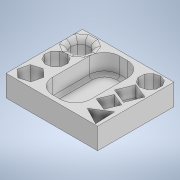
# Autodesk Inventor part: Dice Tower Base
Saved by Autodesk Inventor 2022 (Build 260153000, 153)
## iProperties
Created: 2022-07-25
Part Number: Dice Tower Base
Material: Generic
Document SubType Name: Modeling
Designer: dech3
Density: 1 g/cm^3
Appearance: Default
Author: dech3
Autodesk Inventor part; units mm, degrees
ref_plane "YZ Plane" through (0, 0, 0) normal (1, 0, 0) x (0, 1, 0)
ref_plane "XZ Plane" through (0, 0, 0) normal (0, 1, 0) x (-1, 0, 0)
ref_plane "XY Plane" through (0, 0, 0) normal (0, 0, 1) x (1, 0, 0)
sketch "Sketch1" plane through (0, 0, 0) normal (0, 1, 0) x (-1, 0, 0)
  line L0 (60, -50) -> (-60, -50)
  line L1 (-60, -50) -> (-60, 50)
  line L2 (-60, 50) -> (60, 50)
  line L3 (60, 50) -> (60, -50)
  point P0 (0, 0)
  dimension "d0" = 120
  dimension "d1" = 100
  dimension "d2" = 60
  dimension "d3" = 50
  constraints: 8 end point, 2 parallel, 1 horizontal, 1 perpendicular
  measures "d0" distance between parallel lines of L1 L3
  measures "d1" distance between parallel lines of L2 L0
  measures "d2" distance from line of point (0, 0) L1
  measures "d3" distance from line of point (0, 0) L0
extrude "Extrusion1" add sketch "Sketch1" along normal blind 28
sketch "Sketch2" plane through (0, 28, 0) normal (0, 1, 0) x (1, 0, 0)
  line L0 (-25, 44) -> (25, 44)
  line L1 (25, 44) -> (25, -44)
  line L2 (25, -44) -> (-25, -44)
  line L3 (-25, -44) -> (-25, 44)
  line L4 (60, 50) -> (-60, 50) projected
  line L5 (-60, -50) -> (60, -50) projected
  line L6 (60, -50) -> (60, 50) projected
  line L7 (-60, 50) -> (-60, -50) projected
  dimension "d20" = 6
  dimension "d21" = 6
  dimension "d22" = 35
  dimension "d23" = 35
  constraints: 8 end point, 2 parallel, 1 horizontal, 1 perpendicular
  measures "d20" distance between parallel lines of L0 L4
  measures "d21" distance between parallel lines of L5 L2
  measures "d22" distance between parallel lines of L1 L6
  measures "d23" distance between parallel lines of L7 L3
extrude "Extrusion2" cut sketch "Sketch2" against normal blind 25 contours L0 L1 L2 L3
fillet "Fillet2" radius 20 4 edges at (-25, 15.5, -44) (25, 15.5, -44) (-25, 15.5, 44) (25, 15.5, 44)
fillet "Fillet3" radius 4 8 edges at (19.1421, 3, -38.1421) (25, 3, 0) (19.1421, 3, 38.1421) (0, 3, 44) (-19.1421, 3, 38.1421) (-25, 3, 0) (-19.1421, 3, -38.1421) (0, 3, -44)
sketch "Sketch3" plane through (0, 28, 0) normal (0, 1, 0) x (1, 0, 0)
  line L0 (-30.7335, -30) -> (-33.9026, -43.4891)
  line L1 (-33.9026, -43.4891) -> (-47.1691, -47.4891)
  line L2 (-47.1691, -47.4891) -> (-57.2665, -38)
  line L3 (-57.2665, -38) -> (-54.0974, -24.5109)
  line L4 (-54.0974, -24.5109) -> (-40.8309, -20.5109)
  line L5 (-40.8309, -20.5109) -> (-30.7335, -30)
  line L6 (-60, -50) -> (60, -50) projected
  line L7 (-60, 50) -> (-60, -50) projected
  line L8 (-30.6404, 1.7159) -> (-31.5, -6.3615)
  line L9 (-31.5, -6.3615) -> (-36.9432, -12.391)
  line L10 (-36.9432, -12.391) -> (-44.8909, -14.0695)
  line L11 (-44.8909, -14.0695) -> (-52.3073, -10.7559)
  line L12 (-52.3073, -10.7559) -> (-56.3596, -3.7159)
  line L13 (-56.3596, -3.7159) -> (-55.5, 4.3615)
  line L14 (-55.5, 4.3615) -> (-50.0568, 10.391)
  line L15 (-50.0568, 10.391) -> (-42.1091, 12.0695)
  line L16 (-42.1091, 12.0695) -> (-34.6927, 8.7559)
  line L17 (-34.6927, 8.7559) -> (-30.6404, 1.7159)
  line L18 (-33, 23.6815) -> (-38.6238, 19.0103)
  line L19 (-38.6238, 19.0103) -> (-45.9191, 18.5369)
  line L20 (-45.9191, 18.5369) -> (-52.0995, 22.442)
  line L21 (-52.0995, 22.442) -> (-54.8041, 29.234)
  line L22 (-54.8041, 29.234) -> (-53, 36.3185)
  line L23 (-53, 36.3185) -> (-47.3762, 40.9897)
  line L24 (-47.3762, 40.9897) -> (-40.0809, 41.4631)
  line L25 (-40.0809, 41.4631) -> (-33.9005, 37.558)
  line L26 (-33.9005, 37.558) -> (-31.1959, 30.766)
  line L27 (-31.1959, 30.766) -> (-33, 23.6815)
  line L28 (55, -22.7209) -> (56, -48.7017)
  line L29 (56, -48.7017) -> (33, -36.5774)
  line L30 (33, -36.5774) -> (55, -22.7209)
  line L31 (60, -50) -> (60, 50) projected
  line L32 (35, -3.35) -> (51.6894, -10.0928)
  line L33 (51.6894, -10.0928) -> (44.9466, -26.7821)
  line L34 (44.9466, -26.7821) -> (28.2572, -20.0394)
  line L35 (28.2572, -20.0394) -> (35, -3.35)
  line L36 (38, 21.9687) -> (57.9687, 14)
  line L37 (57.9687, 14) -> (50, -5.9687)
  line L38 (50, -5.9687) -> (30.0313, 2)
  line L39 (30.0313, 2) -> (38, 21.9687)
  line L40 (51, 23.8759) -> (43.1245, 21.8859)
  line L41 (43.1245, 21.8859) -> (35.5835, 24.9051)
  line L42 (35.5835, 24.9051) -> (31.2572, 31.7801)
  line L43 (31.2572, 31.7801) -> (31.7983, 39.8851)
  line L44 (31.7983, 39.8851) -> (37, 46.1241)
  line L45 (37, 46.1241) -> (44.8755, 48.1141)
  line L46 (44.8755, 48.1141) -> (52.4165, 45.0949)
  line L47 (52.4165, 45.0949) -> (56.7428, 38.2199)
  line L48 (56.7428, 38.2199) -> (56.2017, 30.1149)
  line L49 (56.2017, 30.1149) -> (51, 23.8759)
  point P0 (-44, -34)
  point P1 (-43.5, -1)
  point P2 (-43, 30)
  point P3 (48, -36)
  point P4 (40, -15)
  point P5 (53, -20.2983)
  point P6 (44, 8)
  point P7 (44, 35)
  dimension "d24" = 24
  dimension "d25" = 16
  dimension "d26" = 16
  dimension "d27" = 12
  dimension "d28" = 49
  dimension "d29" = 16.5
  dimension "d31" = 25
  dimension "d32" = 4.5
  dimension "d33" = 22.5
  dimension "d34" = 80
  dimension "d35" = 17
  dimension "d37" = 7
  dimension "d38" = 26
  dimension "d39" = 14
  dimension "d40" = 12
  dimension "d42" = 18
  dimension "d43" = 18
  dimension "d44" = 11.65
  dimension "d45" = 9
  dimension "d46" = 25
  dimension "d47" = 35
  dimension "d48" = 20
  dimension "d49" = 21.5
  dimension "d50" = 21.5
  dimension "d52" = 10.75
  dimension "d53" = 10.75
  dimension "d54" = 22
  dimension "d55" = 16
  dimension "d56" = 58
  dimension "d57" = 4
  dimension "d58" = 25
  dimension "d59" = 85
  dimension "d60" = 16
  dimension "d61" = 23
  constraints: 94 end point, 4 parallel, 2 perpendicular, 83 other
  measures "d24" distance between parallel lines of L5 L2
  measures "d25" distance from line of L6 point (-44, -34)
  measures "d26" distance from line of L7 point (-44, -34)
  measures "d27" vertical distance of L6.start L2.end
  measures "d28" distance from line of point (-43.5, -1) L6
  measures "d29" distance from line of L7 point (-43.5, -1)
  measures "d31" distance between parallel lines of L17 L12
  measures "d32" distance from line of L7 L13.end
  measures "d33" distance between parallel lines of L26 L21
  measures "d34" distance from line of L6 point (-43, 30)
  measures "d35" distance from line of L7 point (-43, 30)
  measures "d37" distance from line of L7 L22.end
  measures "d38" distance of L28.start L28.end
  measures "d39" distance from line of L6 point (48, -36)
  measures "d40" distance from line of L31 point (48, -36)
  measures "d42" distance between parallel lines of L33 L35
  measures "d43" distance between parallel lines of L34 L32
  measures "d44" vertical distance of L32.start point (40, -15)
  measures "d45" distance from line of L35 point (40, -15)
  measures "d46" distance from line of L31 L32.start
  measures "d47" distance from line of L6 point (40, -15)
  measures "d48" distance from line of L31 point (40, -15)
  measures "d49" distance between parallel lines of L37 L39
  measures "d50" distance between parallel lines of L38 L36
  measures "d52" distance from line of L39 point (44, 8)
  measures "d53" distance from line of L36 point (44, 8)
  measures "d54" distance from line of L31 L39.end
  measures "d55" distance from line of L31 point (44, 8)
  measures "d56" distance from line of L6 point (44, 8)
  measures "d57" distance from line of L31 L28.end
  measures "d58" distance between parallel lines of L48 L43
  measures "d59" distance from line of L6 point (44, 35)
  measures "d60" distance from line of L31 point (44, 35)
  measures "d61" distance from line of L31 L44.end
extrude "Extrusion3" cut sketch "Sketch3" against normal blind 25
chamfer "Chamfer1" distance 10.5 angle 45 4 edges at (34.0156, 3, -11.9844) (47.9844, 3, -17.9844) (53.9844, 3, -4.0156) (40.0156, 3, 1.9844)
fillet "Fillet4" radius 7 10 edges at (-43.7285, 28, -41.2264) (-50.1881, 28, -38.6541) (-36.9907, 28, -39.5106) (-32.5482, 28, -34.162) (-32.0979, 28, -27.2237) (-35.8119, 28, -21.3459) (-42.2715, 28, -18.7736) (-49.0093, 28, -20.4894) (-53.4518, 28, -25.838) (-53.9021, 28, -32.7763)
equation "\"d2\" = 0.5 * d0"
equation "\"d3\" = 0.5 * d1"
equation "\"d45\" = 0.5 * d42"
body "Solid1"
